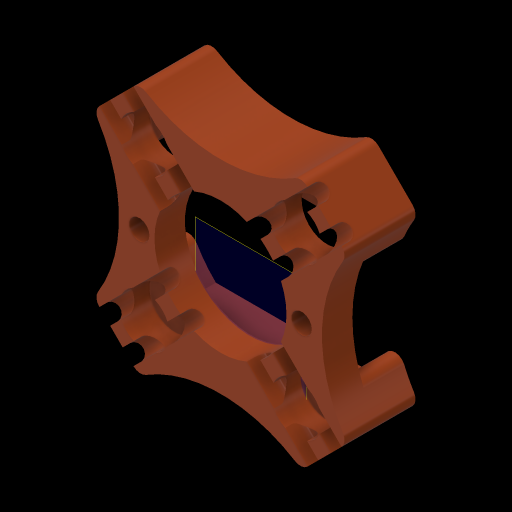
# Autodesk Inventor part: WobbleX WS12 Bottom
Saved by Autodesk Inventor 2023.2 (Build 272271000, 271)
## iProperties
Created: 2023-02-17
Part Number: WobbleX WS12 Bottom
Material: ABS Plastic
Document SubType Name: Modeling
Designer: remop
Density: 1.06 g/cm^3
Appearance: Smooth - Light Orange
Author: remop
Autodesk Inventor part; units mm, degrees
ref_plane "YZ Plane" through (0, 0, 0) normal (1, 0, 0) x (0, 1, 0)
ref_plane "XZ Plane" through (0, 0, 0) normal (0, 1, 0) x (-1, 0, 0)
ref_plane "XY Plane" through (0, 0, 0) normal (0, 0, 1) x (1, 0, 0)
sketch "Sketch1" plane through (0, 0, 0) normal (0, 0, 1) x (1, 0, 0)
  circle A0 centre (-16, 9.3) radius 2
  circle A1 centre (16, 9.3) radius 2
  arc A2 (17.1586, 33.1536) -> (14.6996, 33.4447) centre (15.7444, 31.7393) ccw projected
  arc A3 (-14.6996, 33.4447) -> (14.6996, 33.4447) centre (0, 57.439) ccw projected
  arc A4 (-14.6996, 33.4447) -> (-17.1586, 33.1536) centre (-15.7444, 31.7393) ccw projected
  line L0 (-23.8536, 26.4586) -> (-17.1586, 33.1536) projected
  arc A5 (-23.8536, 26.4586) -> (-24.1447, 23.9996) centre (-22.4393, 25.0444) ccw projected
  arc A6 (-24.1447, -5.3996) -> (-24.1447, 23.9996) centre (-48.139, 9.3) ccw projected
  arc A7 (-24.1447, -5.3996) -> (-23.8536, -7.8586) centre (-22.4393, -6.4444) ccw projected
  line L1 (-17.1586, -14.5536) -> (-23.8536, -7.8586) projected
  arc A8 (-17.1586, -14.5536) -> (-14.6996, -14.8447) centre (-15.7444, -13.1393) ccw projected
  arc A9 (14.6996, -14.8447) -> (-14.6996, -14.8447) centre (0, -38.839) ccw projected
  arc A10 (14.6996, -14.8447) -> (17.1586, -14.5536) centre (15.7444, -13.1393) ccw projected
  line L2 (23.8536, -7.8586) -> (17.1586, -14.5536) projected
  arc A11 (23.8536, -7.8586) -> (24.1447, -5.3996) centre (22.4393, -6.4444) ccw projected
  arc A12 (24.1447, 23.9996) -> (24.1447, -5.3996) centre (48.139, 9.3) ccw projected
  arc A13 (24.1447, 23.9996) -> (23.8536, 26.4586) centre (22.4393, 25.0444) ccw projected
  line L3 (17.1586, 33.1536) -> (23.8536, 26.4586) projected
  circle A14 centre (15, 24.3) radius 5 projected
  circle A15 centre (15, -5.7) radius 5 projected
  circle A16 centre (-15, -5.7) radius 5 projected
  circle A17 centre (-15, 24.3) radius 5 projected
  circle A18 centre (0, 9.3) radius 13 projected
  point P0 (0, 0)
  dimension "d6" = 32
  dimension "d7" = 4
  dimension "d9" = 16
  constraints: 2 centre point, 2 horizontal alignment, 1 equal radius
  measures "d6" distance of A1.centre A0.centre
  measures "d7" diameter of A0
  measures "d9" distance of A0.centre A18.centre
ref_plane "Work Plane1" through (0, 0, 0) normal (0, 0, -1) x (-1, 0, 0)
sketch "Sketch2" plane through (0, 0, 0) normal (0, 0, -1) x (-1, 0, 0)
  line L0 (14.6969, -5.7) -> (-14.6969, -5.7) projected
  arc A0 (14.6969, -5.7) -> (14.6969, 24.3) centre (0, 9.3) ccw projected
  line L1 (-14.6969, 24.3) -> (14.6969, 24.3) projected
  arc A1 (-14.6969, 24.3) -> (-14.6969, -5.7) centre (0, 9.3) ccw projected
  circle A2 centre (0, 9.3) radius 6 projected
  circle A3 centre (-11.3137, -2.0137) radius 2.4 projected
  circle A4 centre (11.3137, -2.0137) radius 2.4 projected
  circle A5 centre (16, 9.3) radius 2.4 projected
  circle A6 centre (11.3137, 20.6137) radius 2.4 projected
  circle A7 centre (-11.3137, 20.6137) radius 2.4 projected
  circle A8 centre (-16, 9.3) radius 2.4 projected
  arc A9 (14.8997, -6.2) -> (14.8997, 24.8) centre (0, 9.3) ccw
  line L2 (14.8997, -6.2) -> (-14.8997, -6.2)
  arc A10 (-14.8997, 24.8) -> (-14.8997, -6.2) centre (0, 9.3) ccw
  line L3 (-14.8997, 24.8) -> (14.8997, 24.8)
  line L4 (-22.9143, 27.3979) -> (-18.0979, 32.2143) projected
  arc A11 (-22.9143, 27.3979) -> (-23.4728, 23.9282) centre (-20.7929, 25.2766) ccw projected
  arc A12 (-23.4728, -5.3282) -> (-23.4728, 23.9282) centre (-52.5447, 9.3) ccw projected
  arc A13 (-23.4728, -5.3282) -> (-22.9143, -8.7979) centre (-20.7929, -6.6766) ccw projected
  line L5 (-18.0979, -13.6143) -> (-22.9143, -8.7979) projected
  arc A14 (-18.0979, -13.6143) -> (-14.6282, -14.1728) centre (-15.9766, -11.4929) ccw projected
  arc A15 (14.6282, -14.1728) -> (-14.6282, -14.1728) centre (0, -43.2447) ccw projected
  arc A16 (14.6282, -14.1728) -> (18.0979, -13.6143) centre (15.9766, -11.4929) ccw projected
  line L6 (22.9143, -8.7979) -> (18.0979, -13.6143) projected
  arc A17 (22.9143, -8.7979) -> (23.4728, -5.3282) centre (20.7929, -6.6766) ccw projected
  arc A18 (23.4728, 23.9282) -> (23.4728, -5.3282) centre (52.5447, 9.3) ccw projected
  arc A19 (23.4728, 23.9282) -> (22.9143, 27.3979) centre (20.7929, 25.2766) ccw projected
  line L7 (18.0979, 32.2143) -> (22.9143, 27.3979) projected
  arc A20 (18.0979, 32.2143) -> (14.6282, 32.7728) centre (15.9766, 30.0929) ccw projected
  arc A21 (-14.6282, 32.7728) -> (14.6282, 32.7728) centre (0, 61.8447) ccw projected
  arc A22 (-14.6282, 32.7728) -> (-18.0979, 32.2143) centre (-15.9766, 30.0929) ccw projected
  circle A23 centre (-15, -5.7) radius 5 projected
  circle A24 centre (15, -5.7) radius 5 projected
  circle A25 centre (15, 24.3) radius 5 projected
  circle A26 centre (-15, 24.3) radius 5 projected
  circle A27 centre (0, 9.3) radius 13 projected
  arc A28 (-14.6996, 33.4447) -> (-17.1586, 33.1536) centre (-15.7444, 31.7393) ccw projected
  arc A29 (-14.6996, 33.4447) -> (14.6996, 33.4447) centre (0, 57.439) ccw projected
  arc A30 (17.1586, 33.1536) -> (14.6996, 33.4447) centre (15.7444, 31.7393) ccw projected
  line L8 (23.8536, 26.4586) -> (17.1586, 33.1536) projected
  arc A31 (24.1447, 23.9996) -> (23.8536, 26.4586) centre (22.4393, 25.0444) ccw projected
  arc A32 (24.1447, 23.9996) -> (24.1447, -5.3996) centre (48.139, 9.3) ccw projected
  arc A33 (23.8536, -7.8586) -> (24.1447, -5.3996) centre (22.4393, -6.4444) ccw projected
  line L9 (17.1586, -14.5536) -> (23.8536, -7.8586) projected
  arc A34 (14.6996, -14.8447) -> (17.1586, -14.5536) centre (15.7444, -13.1393) ccw projected
  arc A35 (14.6996, -14.8447) -> (-14.6996, -14.8447) centre (0, -38.839) ccw projected
  arc A36 (-17.1586, -14.5536) -> (-14.6996, -14.8447) centre (-15.7444, -13.1393) ccw projected
  line L10 (-23.8536, -7.8586) -> (-17.1586, -14.5536) projected
  arc A37 (-24.1447, -5.3996) -> (-23.8536, -7.8586) centre (-22.4393, -6.4444) ccw projected
  arc A38 (-24.1447, -5.3996) -> (-24.1447, 23.9996) centre (-48.139, 9.3) ccw projected
  arc A39 (-23.8536, 26.4586) -> (-24.1447, 23.9996) centre (-22.4393, 25.0444) ccw projected
  line L11 (-17.1586, 33.1536) -> (-23.8536, 26.4586) projected
  circle A40 centre (-15, 24.3) radius 5 projected
  circle A41 centre (-15, -5.7) radius 5 projected
  circle A42 centre (15, -5.7) radius 5 projected
  circle A43 centre (15, 24.3) radius 5 projected
  circle A44 centre (0, 9.3) radius 13 projected
  point P0 (0, 0)
  point P1 (20.5924, 3.119)
  point P2 (-20.5924, 3.119)
  point P3 (-20.5924, 15.481)
  point P4 (20.5924, 15.481)
  point P5 (20.6466, 3.3026)
  point P6 (20.6466, 15.2974)
  point P7 (0, 29.3)
  point P8 (-20.6466, 15.2974)
  point P9 (0, -10.7)
  point P10 (-20.6466, 3.3026)
  dimension "d2" = 0.5
  constraints: 4 end point, 4 point on circle, 2 centre point, 3 other
  measures "d2" distance between parallel lines of L1 L3
extrude "Extrusion2" add sketch "Sketch2" along normal blind 8 contours A23 A10 L2 | L2 A24 A9 A18 A17 L6 A16 A15 A14 L5 A13 A12 A10 A23 | L2 A9 A24 | A12 A13 L10 A37 A38 A10 | A9 A32 A33 L9 A17 A18 | A38 A39 L11 A11 A12 A10 | A12 A11 L4 A22 A21 A20 L7 A19 A18 A9 A25 L3 A26 A10 | A14 A15 A35 A36 L10 | A26 L3 A10 | A9 A18 A19 L8 A31 A32 | A9 L3 A25 | L9 A34 A35 A15 A16 | L11 A28 A29 A21 A22 | A20 A21 A29 A30 L8
extrude "Extrusion3" add sketch "Sketch1" along normal blind 6
fillet "Fillet2" radius 2 4 edges at (20.6466, 3.3026, -4) (20.6466, 15.2974, -4) (-20.6466, 15.2974, -4) (-20.6466, 3.3026, -4)
sketch "Sketch6" plane through (0, 0, 6) normal (0, 0, 1) x (1, 0, 0)
  line L0 (23.8536, 26.4586) -> (17.1586, 33.1536) projected
  arc A0 (17.1586, 33.1536) -> (14.6996, 33.4447) centre (15.7444, 31.7393) ccw projected
  arc A1 (-14.6996, 33.4447) -> (14.6996, 33.4447) centre (0, 57.439) ccw projected
  arc A2 (-14.6996, 33.4447) -> (-17.1586, 33.1536) centre (-15.7444, 31.7393) ccw projected
  line L1 (-17.1586, 33.1536) -> (-23.8536, 26.4586) projected
  arc A3 (-23.8536, 26.4586) -> (-24.1447, 23.9996) centre (-22.4393, 25.0444) ccw projected
  arc A4 (-24.1447, -5.3996) -> (-24.1447, 23.9996) centre (-48.139, 9.3) ccw projected
  arc A5 (-24.1447, -5.3996) -> (-23.8536, -7.8586) centre (-22.4393, -6.4444) ccw projected
  line L2 (-23.8536, -7.8586) -> (-17.1586, -14.5536) projected
  arc A6 (-17.1586, -14.5536) -> (-14.6996, -14.8447) centre (-15.7444, -13.1393) ccw projected
  arc A7 (14.6996, -14.8447) -> (-14.6996, -14.8447) centre (0, -38.839) ccw projected
  arc A8 (14.6996, -14.8447) -> (17.1586, -14.5536) centre (15.7444, -13.1393) ccw projected
  line L3 (17.1586, -14.5536) -> (23.8536, -7.8586) projected
  arc A9 (23.8536, -7.8586) -> (24.1447, -5.3996) centre (22.4393, -6.4444) ccw projected
  arc A10 (24.1447, 23.9996) -> (24.1447, -5.3996) centre (48.139, 9.3) ccw projected
  arc A11 (24.1447, 23.9996) -> (23.8536, 26.4586) centre (22.4393, 25.0444) ccw projected
  circle A12 centre (-16, 9.3) radius 2 projected
  circle A13 centre (16, 9.3) radius 2 projected
  circle A14 centre (0, 9.3) radius 13 projected
  circle A15 centre (-15, 24.3) radius 5 projected
  circle A16 centre (-15, -5.7) radius 5 projected
  circle A17 centre (15, -5.7) radius 5 projected
  circle A18 centre (15, 24.3) radius 5 projected
  line L4 (-4.5702, -1.9877) -> (-18.7123, -16.1298)
  line L5 (-18.7123, -16.1298) -> (-20.8336, -14.0085)
  line L6 (-20.8336, -14.0085) -> (-6.6915, 0.1336)
  line L7 (-6.6915, 0.1336) -> (-4.5702, -1.9877)
  line L8 (-23.8536, -7.8586) -> (-17.1586, -14.5536) projected
  line L9 (-11.2877, 4.7298) -> (-25.4298, -9.4123)
  line L10 (-25.4298, -9.4123) -> (-23.3085, -11.5336)
  line L11 (-23.3085, -11.5336) -> (-9.1664, 2.6085)
  line L12 (-9.1664, 2.6085) -> (-11.2877, 4.7298)
  point P0 (0, 0)
  point P1 (-21.7435, -9.9687)
  point P2 (-19.5493, -7.7745)
  point P3 (-19.4627, -3.4452)
  point P4 (-23.8648, -7.8473)
  point P5 (-17.0745, -10.2493)
  point P6 (-19.2687, -12.4435)
  point P7 (-17.1473, -14.5648)
  point P8 (-12.7452, -10.1627)
  point P9 (-7.8713, -1.0462)
  point P10 (-10.4507, -3.6255)
  point P11 (-10.5373, -7.9548)
  point P12 (-5.198, -2.6156)
  point P13 (-12.9255, -1.1507)
  point P14 (-10.3462, 1.4287)
  point P15 (-11.9156, 4.102)
  point P16 (-17.2548, -1.2373)
  dimension "d39" = 1.75
  dimension "d40" = 1.75
  dimension "d41" = 10
  dimension "d42" = 10
  dimension "d43" = 10
  dimension "d44" = 10
  dimension "d45" = 3
  dimension "d46" = 3
  constraints: 16 end point, 6 parallel, 2 perpendicular
  measures "d39" distance from line of L6 A16.centre
  measures "d40" distance from line of A16.centre L11
  measures "d41" distance from line of L5 A16.centre
  measures "d42" distance from line of A16.centre L7
  measures "d43" distance from line of L12 A16.centre
  measures "d44" distance from line of L10 A16.centre
  measures "d45" distance of L4.end L5.end
  measures "d46" distance of L9.end L10.end
extrude "Extrusion6" cut sketch "Sketch6" against normal blind 3 contours A6 L2 L6 A16 L4 | L9 A16 L11 L2 A5 | A16 L6 A14 L4 | L9 A14 L11 A16
fillet "Fillet5" radius 1.5 8 edges at (-7.8677, -5.2852, 3) (-9.161, -2.3358, 3) (-14.9463, -12.3638, 3) (-18.1716, -11.3464, 3) (-14.5852, 1.4323, 3) (-11.6358, 0.139, 3) (-21.6638, -5.6463, 3) (-20.6464, -8.8716, 3)
pattern_circular "Circular Pattern2" count 4 over 360 about axis through (0, 9.3, 0) along (0, 0, 1) of "Fillet5", "Extrusion6"
equation "\"d9\" = 0.5 * d6"
equation "\"d40\" = d39"
equation "\"d42\" = d41"
equation "\"d43\" = d41"
equation "\"d44\" = d41"
equation "\"d46\" = d45"
body "Solid1"
